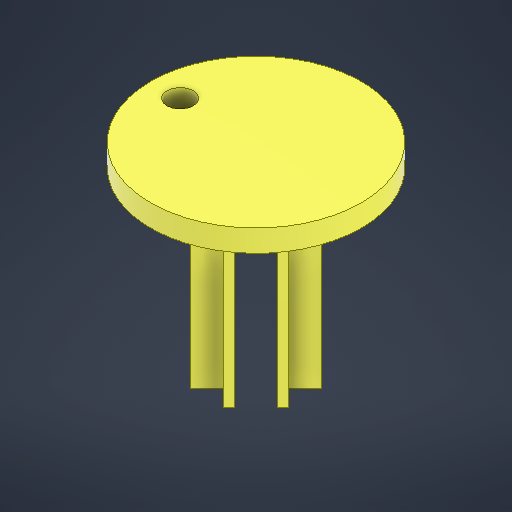
# Autodesk Inventor part: OGPlatform
Saved by Autodesk Inventor 2027 (Build 310192060, 192F)
## iProperties
Created: 2026-07-04
Part Number: OGPlatform
Material: ABS Plastic
Document SubType Name: Modeling
Designer: machnach0
Density: 1.06 g/cm^3
Appearance: Smooth - Yellow
Author: machnach0
Autodesk Inventor part; units mm, degrees
ref_plane "YZ Plane" through (0, 0, 0) normal (1, 0, 0) x (0, 1, 0)
ref_plane "XZ Plane" through (0, 0, 0) normal (0, 1, 0) x (-1, 0, 0)
ref_plane "XY Plane" through (0, 0, 0) normal (0, 0, 1) x (1, 0, 0)
sketch "Sketch1" plane through (0, 0, 0) normal (0, 1, 0) x (-1, 0, 0)
  circle A0 centre (0, 0) radius 30.48
  line L0 (-6.35, 0) -> (-12.7, 6.35)
  line L1 (-12.7, 6.35) -> (-14.2875, 4.7625)
  line L2 (-14.2875, 4.7625) -> (-9.525, 0)
  line L3 (-9.525, 0) -> (-6.35, 0)
  line L4 (-6.35, 0) -> (-12.7, -6.35)
  line L5 (-12.7, -6.35) -> (-14.2875, -4.7625)
  line L6 (-14.2875, -4.7625) -> (-9.525, 0)
  line L7 (0, 30.48) -> (0, -30.48)
  line L8 (0, -6.35) -> (-6.35, -12.7)
  line L9 (-6.35, -12.7) -> (-4.7625, -14.2875)
  line L10 (-4.7625, -14.2875) -> (0, -9.525)
  line L11 (0, -9.525) -> (0, -6.35)
  line L12 (4.7625, -14.2875) -> (0, -9.525)
  line L13 (6.35, -12.7) -> (4.7625, -14.2875)
  line L14 (0, -6.35) -> (6.35, -12.7)
  line L15 (6.35, 0) -> (12.7, -6.35)
  line L16 (12.7, -6.35) -> (14.2875, -4.7625)
  line L17 (14.2875, -4.7625) -> (9.525, 0)
  line L18 (9.525, 0) -> (6.35, 0)
  line L19 (14.2875, 4.7625) -> (9.525, 0)
  line L20 (12.7, 6.35) -> (14.2875, 4.7625)
  line L21 (6.35, 0) -> (12.7, 6.35)
  line L22 (0, 6.35) -> (6.35, 12.7)
  line L23 (6.35, 12.7) -> (4.7625, 14.2875)
  line L24 (4.7625, 14.2875) -> (0, 9.525)
  line L25 (0, 9.525) -> (0, 6.35)
  line L26 (-4.7625, 14.2875) -> (0, 9.525)
  line L27 (-6.35, 12.7) -> (-4.7625, 14.2875)
  line L28 (0, 6.35) -> (-6.35, 12.7)
  circle A1 centre (21.971, 0) radius 3.81
  point P0 (-7.9375, 0)
  point P1 (0, -7.9375)
  point P2 (7.9375, 0)
  point P3 (0, 7.9375)
  dimension "d0" = 60.96
  dimension "d3" = 45
  dimension "d6" = 6.35
  dimension "d7" = 3.175
  dimension "d8" = 6.35
  dimension "d11" = 360
  dimension "d15" = 7.62
  dimension "d16" = 21.971
  constraints: 58 end point, 2 centre point, 2 horizontal alignment, 2 midpoint, 2 perpendicular, 2 point on circle, 2 symmetric about line, 2 vertical, 1 coincident, 1 horizontal, 57 other
  measures "d0" diameter of A0
  measures "d3" angle of L0 L3
  measures "d6" distance of L0.start point (0, 0)
  measures "d7" distance of L2.end L0.start
  measures "d8" horizontal distance of L0.start L0.end
  measures "d15" diameter of A1
  measures "d16" distance of A1.centre point (0, 0)
extrude "Extrusion1" add sketch "Sketch1" along normal blind 6.35 contours A0 L7 L12 L13 L14 L22 L23 L24 | L7 L26 L27 L28 L8 L9 L10 A0 | L24 L23 L22 L7 | L7 L28 L27 L26 | L10 L9 L8 L7 | L7 L14 L13 L12 | L3 L2 L1 L0 | L4 L5 L6 L3 | L18 L17 L16 L15 | L21 L20 L19 L18 | A1
extrude "Extrusion2" add sketch "Sketch1" against normal blind 50.8 contours L24 L23 L22 L7 | L7 L28 L27 L26 | L10 L9 L8 L7 | L7 L14 L13 L12 | L3 L2 L1 L0 | L4 L5 L6 L3 | L18 L17 L16 L15 | L21 L20 L19 L18
extrude "Extrusion3" cut sketch "Sketch1" along normal blind 6.35 contours A1
body "Solid1"
